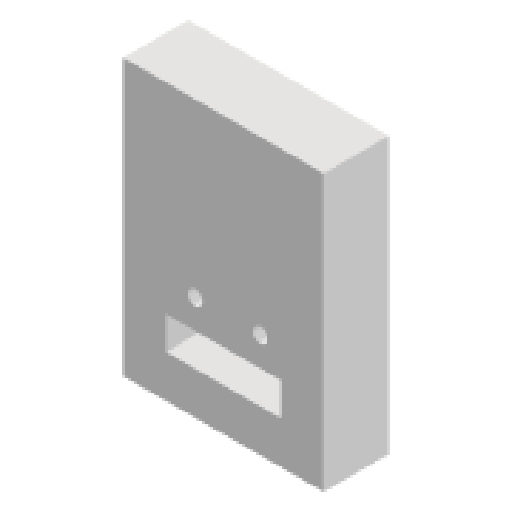
# Autodesk Inventor part: sensor_estructura
Saved by Autodesk Inventor 2025 (Build 290162000, 162)
## iProperties
Created: 2026-02-02
Part Number: sensor_estructura
Material: Genérico
Document SubType Name: Modeling
Designer: HP
Density: 1 g/cm^3
Appearance: Valor por defecto
Author: HP
Autodesk Inventor part; units mm, degrees
ref_plane "YZ Plane" through (0, 0, 0) normal (1, 0, 0) x (0, 1, 0)
ref_plane "XZ Plane" through (0, 0, 0) normal (0, 1, 0) x (-1, 0, 0)
ref_plane "XY Plane" through (0, 0, 0) normal (0, 0, 1) x (1, 0, 0)
sketch "Boceto4" plane through (0, 0, 0) normal (0, 0, 1) x (1, 0, 0)
  circle A0 centre (-1.0562, 12.2493) radius 5 projected
  line L0 (33.4438, -22.7507) -> (-36.5562, -22.7507) projected
  line L1 (33.4438, 47.2493) -> (33.4438, -22.7507) projected
  line L2 (-36.5562, 47.2493) -> (33.4438, 47.2493) projected
  line L3 (-36.5562, -22.7507) -> (-36.5562, 47.2493) projected
  circle A1 centre (21.3438, 12.2493) radius 3.7 projected
  circle A2 centre (-23.4562, 12.2493) radius 3.7 projected
  line L4 (36.4438, 50.2493) -> (-39.5562, 50.2493) projected
  line L5 (-39.5562, 50.2493) -> (-39.5562, -25.7507) projected
  line L6 (-39.5562, -25.7507) -> (36.4438, -25.7507) projected
  line L7 (36.4438, -25.7507) -> (36.4438, 50.2493) projected
  line L8 (33.4438, -22.7507) -> (-36.5562, -22.7507) projected
  line L9 (-36.5562, -22.7507) -> (-36.5562, 47.2493) projected
  line L10 (-36.5562, 47.2493) -> (33.4438, 47.2493) projected
  line L11 (33.4438, 47.2493) -> (33.4438, -22.7507) projected
  point P0 (0, 0)
extrude "Extrusión4" add sketch "Boceto4" against normal blind 10 contours L7 L6 L5 L4
